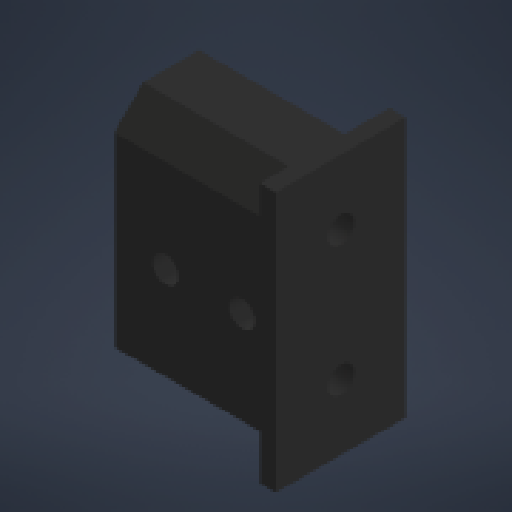
# Autodesk Inventor part: TUBE_PLUGS
Saved by Autodesk Inventor 2026.2 (Build 302298010, 298A)
## iProperties
Created: 2026-04-02
Part Number: TUBE_PLUGS
Material: 3D Print Material - chopped carbon Nylon12 (preferred)
Document SubType Name: Modeling
Designer: 4aida
Density: 1.05184 g/cm^3
Appearance: Black
Mass: 38.5401 g
Surface Area: 96.3872 cm^2
Volume: 36.6408 cm^3
Author: 4aida
Autodesk Inventor part; units mm, degrees
ref_plane "YZ Plane" through (0, 0, 0) normal (1, 0, 0) x (0, 1, 0)
ref_plane "XZ Plane" through (0, 0, 0) normal (0, 1, 0) x (-1, 0, 0)
ref_plane "XY Plane" through (0, 0, 0) normal (0, 0, 1) x (1, 0, 0)
sketch "Sketch1" plane through (0, 0, 0) normal (1, 0, 0) x (0, 1, 0)
  line L0 (-23.8125, -11.1125) -> (23.8125, -11.1125)
  line L1 (23.8125, -11.1125) -> (23.8125, 11.1125)
  line L2 (23.8125, 11.1125) -> (-23.8125, 11.1125)
  line L3 (-23.8125, 11.1125) -> (-23.8125, -11.1125)
  line L4 (-23.8125, -11.1125) -> (23.8125, 11.1125) construction
  line L5 (23.8125, -11.1125) -> (-23.8125, 11.1125) construction
  line L6 (23.8125, 5.4556) -> (18.1556, 11.1125)
  line L7 (-18.1556, 11.1125) -> (-23.8125, 5.4556)
  line L8 (-18.1556, -11.1125) -> (-23.8125, -5.4556)
  line L9 (18.1556, -11.1125) -> (23.8125, -5.4556)
  point P0 (0, 0)
  dimension "d0" = 135
  dimension "d1" = 135
  dimension "d2" = 4
  dimension "d3" = 47.625
  dimension "d4" = 22.225
  constraints: 20 end point, 8 point on line, 4 parallel, 4 perpendicular, 2 midpoint, 1 horizontal
  measures "d0" angle of L2 L6
  measures "d1" angle of L0 L9
  measures "d2" distance from line of L1.end L6
  measures "d3" distance between parallel lines of L3 L1
  measures "d4" distance of L0.end L1.end
extrude "Extrusion1" add sketch "Sketch1" along normal blind 36 contours L8 L3 L7 L2 L6 L1 L9 L0
sketch "Sketch2" plane through (36, 0, 0) normal (1, 0, 0) x (0, 0, -1)
  line L0 (0, 12.7) -> (0, -12.7)
  point P0 (0, 0)
  point P1 (0, 0)
  dimension "d7" = 25.4
  constraints: 3 coincident, 2 end point, 1 midpoint, 1 vertical
  measures "d7" distance of L0.start L0.end
hole "Hole1" at (36, 12.7, 0) at (36, -12.7, 0) direction (-1, 0, 0) diameter 5.105 end through all clearance for "Flat Head Machine Screw (82)" size "#10" standard "Ansi Unified Screw Threads"
sketch "Sketch3" plane through (0, 0, 0) normal (-1, 0, 0) x (0, 0, 1)
  circle A0 centre (0, 12.7) radius 2.5525 projected
  line L0 (-4.7752, 15.457) -> (0, 18.2139)
  line L1 (0, 18.2139) -> (4.7752, 15.457)
  line L2 (4.7752, 15.457) -> (4.7752, 9.943)
  line L3 (4.7752, 9.943) -> (0, 7.1861)
  line L4 (0, 7.1861) -> (-4.7752, 9.943)
  line L5 (-4.7752, 9.943) -> (-4.7752, 15.457)
  circle A1 centre (0, -12.7) radius 2.5525 projected
  line L6 (-4.7752, -9.943) -> (0, -7.1861)
  line L7 (0, -7.1861) -> (4.7752, -9.943)
  line L8 (4.7752, -9.943) -> (4.7752, -15.457)
  line L9 (4.7752, -15.457) -> (0, -18.2139)
  line L10 (0, -18.2139) -> (-4.7752, -15.457)
  line L11 (-4.7752, -15.457) -> (-4.7752, -9.943)
  point P0 (0, 0)
  dimension "d15" = 9.5504
  dimension "d16" = 9.5504
  constraints: 24 end point, 2 coincident, 2 vertical, 26 other
  measures "d15" distance between parallel lines of L3 L0
  measures "d16" distance between parallel lines of L8 L11
extrude "Extrusion2" cut sketch "Sketch3" against normal blind 6.35 contours A0 | L0 L1 L2 L3 L4 L5 | A1 | L6 L7 L8 L9 L10 L11
sketch "Sketch4" plane through (36, 0, 0) normal (1, 0, 0) x (0, 0, -1)
  line L0 (12.7, -25.4) -> (-12.7, -25.4)
  line L1 (-12.7, -25.4) -> (-12.7, 25.4)
  line L2 (-12.7, 25.4) -> (12.7, 25.4)
  line L3 (12.7, 25.4) -> (12.7, -25.4)
  line L4 (12.7, -25.4) -> (-12.7, 25.4) construction
  line L5 (-12.7, -25.4) -> (12.7, 25.4) construction
  circle A0 centre (0, 12.7) radius 2.5525 projected
  circle A1 centre (0, -12.7) radius 2.5525 projected
  point P0 (0, 0)
  dimension "d19" = 25.4
  dimension "d20" = 50.8
  constraints: 12 end point, 2 midpoint, 2 parallel, 1 horizontal, 1 perpendicular
  measures "d19" distance of L1.end L2.end
  measures "d20" distance of L0.end L1.end
extrude "Extrusion3" add sketch "Sketch4" along normal blind 3.175
sketch "Sketch5" plane through (0, -18.1556, 11.1125) normal (0, 0, 1) x (1, 0, 0)
  line L0 (36, 43.5556) -> (36, -7.2444) projected
  line L1 (0, 36.3113) -> (0, 0) projected
  point P0 (0, 18.1556)
  point P1 (31, 18.1556)
  point P2 (5.6, 18.1556)
  point P3 (0, 18.1556)
  dimension "d23" = 25.4
  dimension "d24" = 5
  constraints: 2 horizontal alignment, 1 midpoint
  measures "d23" distance of point (5.6, 18.156) point (31, 18.156)
  measures "d24" distance from line of L0 point (31, 18.156)
hole "Hole2" at (31, 0, 11.1125) at (5.6, 0, 11.1125) direction (0, 0, -1) diameter 5.105 end through all clearance for "Flat Head Machine Screw (82)" size "#10" standard "Ansi Unified Screw Threads"
equation "\"d1\" = d0"
equation "\"d16\" = d15"
body "Solid1"
